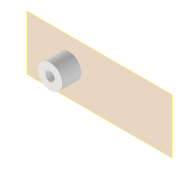
# Autodesk Inventor part: 20_Cube_Insert_Lightsheet_FEPTube_Rotating_hollomotor_driver_v0
Saved by Autodesk Inventor 2022 (Build 260153000, 153)
## iProperties
Created: 2022-04-18
Part Number: 20_Cube_Insert_Lightsheet_FEPTube_Rotating_hollomotor_driver_v0
Material: Generic
Document SubType Name: Modeling
Designer: Prakash Lab
Density: 1 g/cm^3
Appearance: Default
Author: Prakash Lab
Autodesk Inventor part; units mm, degrees
ref_plane "YZ Plane" through (0, 0, 0) normal (1, 0, 0) x (0, 1, 0)
ref_plane "XZ Plane" through (0, 0, 0) normal (0, 1, 0) x (-1, 0, 0)
ref_plane "XY Plane" through (0, 0, 0) normal (0, 0, 1) x (1, 0, 0)
ref_plane "Work Plane1" through (0, 0, 0) normal (0, 0, 1) x (1, 0, 0)
sketch "Sketch1" plane through (0, 0, 0) normal (0, 0, 1) x (1, 0, 0)
  circle A0 centre (15, 1) radius 1.8 projected
  circle A1 centre (15, 1) radius 2 projected
  circle A2 centre (33.5, -2.875) radius 5.0649 projected
  circle A3 centre (15, 1) radius 5.0649
  point P0 (0, 0)
  constraints: 1 centre point, 1 coincident, 1 equal radius
extrude "Extrusion1" add sketch "Sketch1" along normal blind 8 contours A3
ref_plane "Work Plane2" through (23.5, 1, -28) normal (0, -1, 0) x (0, 0, 1)
sketch "Sketch2" plane through (23.5, 1, -28) normal (0, -1, 0) x (0, 0, 1)
  arc A0 (30.1735, -5.6017) -> (31.6642, -5.6017) centre (30.9188, -4.9351) ccw
  circle A1 centre (30.9188, 13.464) radius 1
  line L0 (26.4, 8.5) -> (37.6, 8.5) projected
  point P0 (28, 23.5)
  constraints: 2 centre point, 2 point on circle, 1 equal radius, 4 other
revolve "Revolution1" cut sketch "Sketch2" angle 360 about axis through (15, 1, 0) along (0, 0, 1)
fillet "Fillet1" radius 2 4 edges at (15, -4.0649, 3.9137) (15, 6.0649, 3.9137) (15, -4.0649, 1.9239) (15, 6.0649, 1.9239)
body "Solid1"
